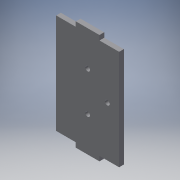
# Autodesk Inventor part: Camera cross bar
Saved by Autodesk Inventor 2018 (Build 220112000, 112)
## iProperties
Created: 2018-05-02
Part Number: Camera cross bar
Material: Generic
Document SubType Name: Modeling
Designer: Ajith Thomas
Density: 1 g/cm^3
Appearance: Default
Author: Ajith Thomas
Autodesk Inventor part; units mm, degrees
ref_plane "YZ Plane" through (0, 0, 0) normal (1, 0, 0) x (0, 1, 0)
ref_plane "XZ Plane" through (0, 0, 0) normal (0, 1, 0) x (-1, 0, 0)
ref_plane "XY Plane" through (0, 0, 0) normal (0, 0, 1) x (1, 0, 0)
sketch "Sketch1" plane through (0, 0, 0) normal (0, 0, 1) x (1, 0, 0)
  line L0 (0, 0) -> (-15, 0) construction
  line L1 (0, 0) -> (0, 3)
  line L2 (-15, 3) -> (0, 3)
  line L3 (-15, 0) -> (-15, 3)
  line L4 (-27.5, 0) -> (-7.5, 0)
  line L5 (6.5, 0) -> (12.5, 0)
  line L6 (6.5, 0) -> (3.5, 0)
  line L7 (-7.5, 0) -> (3.5, 0)
  line L8 (3.5, 8.25) -> (6.5, 8.25) construction
  line L9 (3.5, -71.75) -> (6.5, -71.75) construction
  line L10 (5, 8.25) -> (5, -71.75) construction
  line L11 (-27.5, 0) -> (-27.5, -31.75)
  line L12 (12.5, 0) -> (12.5, -31.75)
  line L13 (-27.5, -31.75) -> (12.5, -31.75) construction
  line L14 (-27.5, 0) -> (-15, 0)
  line L15 (-15, 0) -> (-15, 3)
  line L16 (-15, 3) -> (0, 3)
  line L17 (0, 3) -> (0, 0)
  line L18 (0, 0) -> (12.5, 0)
  line L19 (0, -63.5) -> (0, -66.5)
  line L20 (-15, -66.5) -> (0, -66.5)
  line L21 (-15, -63.5) -> (-15, -66.5)
  line L22 (-27.5, -63.5) -> (-27.5, -31.75)
  line L23 (12.5, -63.5) -> (12.5, -31.75)
  line L24 (-27.5, -63.5) -> (-15, -63.5)
  line L25 (0, -63.5) -> (12.5, -63.5)
  line L26 (0, 0) -> (-15, 0)
extrude "Extrusion1" add sketch "Sketch1" along normal blind 3
sketch "Sketch2" plane through (0, 0, 3) normal (0, 0, 1) x (1, 0, 0)
  line L0 (0, 0) -> (0, 3) projected
  line L1 (0, 3) -> (-15, 3) projected
  line L2 (-15, 3) -> (-15, 0) projected
  line L3 (-15, 0) -> (-27.5, 0) projected
  line L4 (-27.5, 0) -> (-27.5, -63.5) projected
  line L5 (-27.5, -63.5) -> (-15, -63.5) projected
  line L6 (-15, -63.5) -> (-15, -66.5) projected
  line L7 (-15, -66.5) -> (0, -66.5) projected
  line L8 (0, -66.5) -> (0, -63.5) projected
  line L9 (0, -63.5) -> (12.5, -63.5) projected
  line L10 (12.5, -63.5) -> (12.5, 0) projected
  line L11 (12.5, 0) -> (0, 0) projected
  line L12 (0, 3) -> (-15, 3) construction
  line L13 (-7.5, 3) -> (-7.5, -66.5) construction
  line L14 (-15, -66.5) -> (0, -66.5) construction
  line L15 (12.5, -63.5) -> (12.5, 0) construction
  line L16 (12.5, -31.75) -> (-27.5, -31.75) construction
  line L17 (-27.5, 0) -> (-27.5, -63.5) construction
  circle A0 centre (-7.5, -19.25) radius 1.5
  circle A1 centre (5, -31.75) radius 1.5
  circle A2 centre (-7.5, -44.25) radius 1.5
  dimension "d5" = 3
  dimension "d6" = 3
  dimension "d7" = 12.5
  dimension "d8" = 12.5
  constraints: 4 end point, 4 midpoint, 3 centre point, 2 point on line, 1 symmetric about line, 1 other
  measures "d5" diameter of A0
  measures "d6" diameter of A1
  measures "d7" distance from line of L16 A0.centre
  measures "d8" distance from line of L13 A1.centre
extrude "Extrusion2" cut sketch "Sketch2" against normal blind 3 contours A0 | A1 | A2
body "Solid1"
